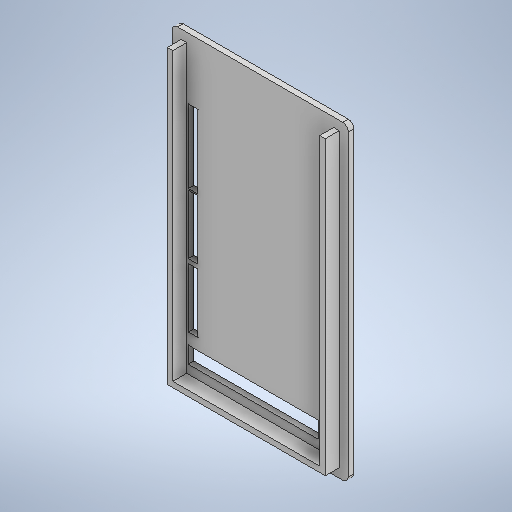
# Autodesk Inventor part: arduino_lid
Saved by Autodesk Inventor 2025 (Build 290162000, 162)
## iProperties
Created: 2025-03-25
Part Number: arduino_lid
Material: Všeobecné
Document SubType Name: Modeling
Designer: lukas
Density: 1 g/cm^3
Appearance: Výchozí
Author: lukas
## iProperties of the stored document arduino_lid_3D tisk.ipt
Created: 2025-03-25
Part Number: arduino_lid_3D tisk
Material: Všeobecné
Document SubType Name: Modeling
Designer: lukas
Density: 1 g/cm^3
Appearance: Výchozí
Author: lukas
Autodesk Inventor part; units mm, degrees
ref_plane "YZ Plane" through (0, 0, 0) normal (1, 0, 0) x (0, 1, 0)
ref_plane "XZ Plane" through (0, 0, 0) normal (0, 1, 0) x (-1, 0, 0)
ref_plane "XY Plane" through (0, 0, 0) normal (0, 0, 1) x (1, 0, 0)
sketch "Náčrt1" plane through (0, 0, 0) normal (0, 1, 0) x (-1, 0, 0)
  line L0 (-6.677663, 17.076554) -> (49.20234, 17.076554)
  line L1 (-9.217661, 14.536556) -> (-9.217661, -88.33345)
  line L2 (-6.677663, -90.873447) -> (49.20234, -90.873447)
  line L3 (51.742337, 14.536556) -> (51.742337, -88.33345)
  line L4 (47.105338, -3.131448) -> (47.105338, -74.251447)
  line L5 (43.679337, -3.131448) -> (47.105338, -3.131448)
  line L6 (43.679337, -29.547447) -> (43.679337, -3.131448)
  line L7 (43.679337, -29.547447) -> (47.105338, -29.547447)
  line L8 (43.679337, -30.055447) -> (47.105338, -30.055447)
  line L9 (43.679337, -51.391447) -> (43.679337, -30.055447)
  line L10 (47.105338, -51.391447) -> (43.679337, -51.391447)
  line L11 (43.679337, -52.915447) -> (47.105338, -52.915447)
  line L12 (43.679337, -74.251447) -> (43.679337, -52.915447)
  line L13 (47.105338, -74.251447) -> (43.679337, -74.251447)
  line L14 (0.434339, -78.380447) -> (47.170339, -78.380447)
  line L15 (47.170339, -84.346448) -> (47.170339, -78.380447)
  line L16 (47.170339, -84.346448) -> (0.434339, -84.346448)
  line L17 (0.434339, -84.346448) -> (0.434339, -78.380447)
  line L18 (-1.154661, -57.995446) -> (-1.154661, -79.331446)
  line L19 (-4.580662, -79.331446) -> (-4.580662, -12.275449)
  line L20 (-1.154661, -79.331446) -> (-4.580662, -79.331446)
  line L21 (-4.580662, -57.995446) -> (-1.154661, -57.995446)
  line L22 (-1.154661, -56.471446) -> (-4.580662, -56.471446)
  line L23 (-1.154661, -35.135447) -> (-1.154661, -56.471446)
  line L24 (-4.580662, -35.135447) -> (-1.154661, -35.135447)
  line L25 (-1.154661, -33.611447) -> (-4.580662, -33.611447)
  line L26 (-1.154661, -12.275449) -> (-1.154661, -33.611447)
  line L27 (-4.580662, -12.275449) -> (-1.154661, -12.275449)
  circle A0 centre (-6.686866, -88.348377) radius 2.522363
  circle A1 centre (49.198008, -88.332369) radius 2.54409
  circle A2 centre (49.211542, 14.551484) radius 2.522363
  circle A3 centre (-6.692632, 14.545779) radius 2.522319
  line L28 (51.742337, 17.076554) -> (-9.217661, 17.076554)
  line L29 (-9.217661, 17.076554) -> (-9.217661, -90.873447)
  line L30 (-9.217661, -90.873447) -> (51.742337, -90.873447)
  line L31 (51.742337, -90.873447) -> (51.742337, 17.076554)
  line L32 (-1.154661, -12.275449) -> (-4.580662, -12.275449)
  line L33 (-4.580662, -12.275449) -> (-4.580662, -33.611447)
  line L34 (-4.580662, -33.611447) -> (-1.154661, -33.611447)
  line L35 (-1.154661, -33.611447) -> (-1.154661, -12.275449)
  line L36 (-4.580662, -35.135447) -> (-1.154661, -35.135447)
  line L37 (-1.154661, -35.135447) -> (-1.154661, -56.471446)
  line L38 (-1.154661, -56.471446) -> (-4.580662, -56.471446)
  line L39 (-4.580662, -56.471446) -> (-4.580662, -35.135447)
  line L40 (-4.580662, -57.995446) -> (-1.154661, -57.995446)
  line L41 (-1.154661, -57.995446) -> (-1.154661, -79.331446)
  line L42 (-1.154661, -79.331446) -> (-4.580662, -79.331446)
  line L43 (-4.580662, -79.331446) -> (-4.580662, -57.995446)
  line L44 (0.434339, -84.346448) -> (47.170339, -84.346448)
  line L45 (47.170339, -84.346448) -> (47.170339, -78.380447)
  line L46 (47.170339, -78.380447) -> (0.434339, -78.380447)
  line L47 (0.434339, -78.380447) -> (0.434339, -84.346448)
  line L48 (43.679337, -74.251447) -> (47.105338, -74.251447)
  line L49 (47.105338, -74.251447) -> (47.105338, -52.915447)
  line L50 (47.105338, -52.915447) -> (43.679337, -52.915447)
  line L51 (43.679337, -52.915447) -> (43.679337, -74.251447)
  line L52 (47.105338, -30.055447) -> (43.679337, -30.055447)
  line L53 (43.679337, -30.055447) -> (43.679337, -51.391447)
  line L54 (43.679337, -51.391447) -> (47.105338, -51.391447)
  line L55 (47.105338, -51.391447) -> (47.105338, -30.055447)
  line L56 (43.679337, -29.547447) -> (47.105338, -29.547447)
  line L57 (47.105338, -29.547447) -> (47.105338, -3.131448)
  line L58 (47.105338, -3.131448) -> (43.679337, -3.131448)
  line L59 (43.679337, -3.131448) -> (43.679337, -29.547447)
  point P0 (0, 0)
  dimension "d0" = 0
  dimension "d1" = 0
  dimension "d2" = 0
  dimension "d3" = 0
  constraints: 64 end point, 16 parallel, 8 horizontal, 8 perpendicular
  measures "d0" distance between parallel lines of L0 L28
  measures "d1" distance between parallel lines of L3 L31
  measures "d2" distance between parallel lines of L30 L2
  measures "d3" distance between parallel lines of L1 L29
sketch "Náčrt1 outline for Vysunutí1" plane through (0, 0, 0) normal (0, 1, 0) x (-1, 0, 0)
  line L0 (51.742337, 14.536556) -> (51.742337, 17.076554)
  line L1 (51.742337, -88.33345) -> (51.742337, 14.536556)
  line L2 (51.742337, 17.076554) -> (49.20234, 17.076554)
  line L3 (51.742337, -90.873447) -> (51.742337, -88.33345)
  line L4 (49.20234, 17.076554) -> (-6.677663, 17.076554)
  line L5 (49.20234, -90.873447) -> (51.742337, -90.873447)
  line L6 (-6.677663, 17.076554) -> (-9.217661, 17.076554)
  line L7 (-6.677663, -90.873447) -> (49.20234, -90.873447)
  line L8 (-9.217661, 17.076554) -> (-9.217661, 14.536556)
  line L9 (-9.217661, -90.873447) -> (-6.677663, -90.873447)
  line L10 (-9.217661, 14.536556) -> (-9.217661, -88.33345)
  line L11 (-9.217661, -88.33345) -> (-9.217661, -90.873447)
  line L12 (-4.580662, -57.995446) -> (-1.154661, -57.995446)
  line L13 (-4.580662, -79.331446) -> (-4.580662, -57.995446)
  line L14 (-1.154661, -79.331446) -> (-4.580662, -79.331446)
  line L15 (-1.154661, -57.995446) -> (-1.154661, -79.331446)
  line L16 (-4.580662, -56.471446) -> (-4.580662, -35.135447)
  line L17 (-1.154661, -56.471446) -> (-4.580662, -56.471446)
  line L18 (-1.154661, -35.135447) -> (-1.154661, -56.471446)
  line L19 (-4.580662, -35.135447) -> (-1.154661, -35.135447)
  line L20 (0.434339, -84.346448) -> (0.434339, -78.380447)
  line L21 (47.170339, -84.346448) -> (0.434339, -84.346448)
  line L22 (47.170339, -78.380447) -> (47.170339, -84.346448)
  line L23 (0.434339, -78.380447) -> (47.170339, -78.380447)
  line L24 (47.105338, -52.915447) -> (47.105338, -74.251447)
  line L25 (43.679337, -52.915447) -> (47.105338, -52.915447)
  line L26 (43.679337, -74.251447) -> (43.679337, -52.915447)
  line L27 (47.105338, -74.251447) -> (43.679337, -74.251447)
  line L28 (-4.580662, -33.611447) -> (-4.580662, -12.275449)
  line L29 (-1.154661, -33.611447) -> (-4.580662, -33.611447)
  line L30 (-1.154661, -12.275449) -> (-1.154661, -33.611447)
  line L31 (-4.580662, -12.275449) -> (-1.154661, -12.275449)
  line L32 (47.105338, -30.055447) -> (47.105338, -51.391447)
  line L33 (43.679337, -30.055447) -> (47.105338, -30.055447)
  line L34 (43.679337, -51.391447) -> (43.679337, -30.055447)
  line L35 (47.105338, -51.391447) -> (43.679337, -51.391447)
  line L36 (47.105338, -29.547447) -> (43.679337, -29.547447)
  line L37 (47.105338, -3.131448) -> (47.105338, -29.547447)
  line L38 (43.679337, -3.131448) -> (47.105338, -3.131448)
  line L39 (43.679337, -29.547447) -> (43.679337, -3.131448)
extrude "Vysunutí1" add sketch "Náčrt1 outline for Vysunutí1" along normal blind 2
sketch "Náčrt2" plane through (0, 2, 0) normal (0, 1, 0) x (1, 0, 0)
  line L0 (-51.742337, -17.076554) -> (9.217661, -17.076554)
  line L1 (9.217661, -17.076554) -> (9.217661, 90.873447)
  line L2 (9.217661, 90.873447) -> (-51.742337, 90.873447)
  line L3 (-51.742337, 90.873447) -> (-51.742337, -17.076554)
  line L4 (-47.105338, 29.547447) -> (-43.679337, 29.547447)
  line L5 (-43.679337, 29.547447) -> (-43.679337, 3.131448)
  line L6 (-43.679337, 3.131448) -> (-47.105338, 3.131448)
  line L7 (-47.105338, 3.131448) -> (-47.105338, 29.547447)
  line L8 (-47.105338, 30.055447) -> (-47.105338, 51.391447)
  line L9 (-47.105338, 51.391447) -> (-43.679337, 51.391447)
  line L10 (-43.679337, 51.391447) -> (-43.679337, 30.055447)
  line L11 (-43.679337, 30.055447) -> (-47.105338, 30.055447)
  line L12 (4.580662, 57.995446) -> (1.154661, 57.995446)
  line L13 (1.154661, 57.995446) -> (1.154661, 79.331446)
  line L14 (1.154661, 79.331446) -> (4.580662, 79.331446)
  line L15 (4.580662, 79.331446) -> (4.580662, 57.995446)
  line L16 (4.580662, 56.471446) -> (4.580662, 35.135447)
  line L17 (4.580662, 35.135447) -> (1.154661, 35.135447)
  line L18 (1.154661, 35.135447) -> (1.154661, 56.471446)
  line L19 (1.154661, 56.471446) -> (4.580662, 56.471446)
  line L20 (4.580662, 33.611447) -> (4.580662, 12.275449)
  line L21 (4.580662, 12.275449) -> (1.154661, 12.275449)
  line L22 (1.154661, 12.275449) -> (1.154661, 33.611447)
  line L23 (1.154661, 33.611447) -> (4.580662, 33.611447)
  line L24 (-0.434339, 84.346448) -> (-0.434339, 78.380447)
  line L25 (-0.434339, 78.380447) -> (-47.170339, 78.380447)
  line L26 (-47.170339, 78.380447) -> (-47.170339, 84.346448)
  line L27 (-47.170339, 84.346448) -> (-0.434339, 84.346448)
  line L28 (-47.105338, 52.915447) -> (-47.105338, 74.251447)
  line L29 (-47.105338, 74.251447) -> (-43.679337, 74.251447)
  line L30 (-43.679337, 74.251447) -> (-43.679337, 52.915447)
  line L31 (-43.679337, 52.915447) -> (-47.105338, 52.915447)
  line L32 (-52.742337, -18.076554) -> (10.217661, -18.076554)
  line L33 (10.217661, -18.076554) -> (10.217661, 91.873447)
  line L34 (10.217661, 91.873447) -> (-52.742337, 91.873447)
  line L35 (-52.742337, 91.873447) -> (-52.742337, -18.076554)
  point P0 (0, 0)
  dimension "d6" = 1
  constraints: 8 end point, 3 other
  measures "d6" distance between parallel lines of L3 L35
extrude "Vysunutí2" add sketch "Náčrt2" against normal up to surface (2 mm away) contours L35 L34 L33 L32
sketch "Náčrt3" plane through (0, 2, 0) normal (0, 1, 0) x (1, 0, 0)
  line L0 (10.217661, -18.076554) -> (10.217661, 91.873447)
  line L1 (10.217661, 91.873447) -> (-52.742337, 91.873447)
  line L2 (-52.742337, 91.873447) -> (-52.742337, -18.076554)
  line L3 (-52.742337, -18.076554) -> (10.217661, -18.076554)
  line L4 (-47.105338, 29.547447) -> (-43.679337, 29.547447)
  line L5 (-43.679337, 29.547447) -> (-43.679337, 3.131448)
  line L6 (-43.679337, 3.131448) -> (-47.105338, 3.131448)
  line L7 (-47.105338, 3.131448) -> (-47.105338, 29.547447)
  line L8 (-47.105338, 30.055447) -> (-47.105338, 51.391447)
  line L9 (-47.105338, 51.391447) -> (-43.679337, 51.391447)
  line L10 (-43.679337, 51.391447) -> (-43.679337, 30.055447)
  line L11 (-43.679337, 30.055447) -> (-47.105338, 30.055447)
  line L12 (4.580662, 57.995446) -> (1.154661, 57.995446)
  line L13 (1.154661, 57.995446) -> (1.154661, 79.331446)
  line L14 (1.154661, 79.331446) -> (4.580662, 79.331446)
  line L15 (4.580662, 79.331446) -> (4.580662, 57.995446)
  line L16 (4.580662, 56.471446) -> (4.580662, 35.135447)
  line L17 (4.580662, 35.135447) -> (1.154661, 35.135447)
  line L18 (1.154661, 35.135447) -> (1.154661, 56.471446)
  line L19 (1.154661, 56.471446) -> (4.580662, 56.471446)
  line L20 (4.580662, 33.611447) -> (4.580662, 12.275449)
  line L21 (4.580662, 12.275449) -> (1.154661, 12.275449)
  line L22 (1.154661, 12.275449) -> (1.154661, 33.611447)
  line L23 (1.154661, 33.611447) -> (4.580662, 33.611447)
  line L24 (-0.434339, 84.346448) -> (-0.434339, 78.380447)
  line L25 (-0.434339, 78.380447) -> (-47.170339, 78.380447)
  line L26 (-47.170339, 78.380447) -> (-47.170339, 84.346448)
  line L27 (-47.170339, 84.346448) -> (-0.434339, 84.346448)
  line L28 (-47.105338, 52.915447) -> (-47.105338, 74.251447)
  line L29 (-47.105338, 74.251447) -> (-43.679337, 74.251447)
  line L30 (-43.679337, 74.251447) -> (-43.679337, 52.915447)
  line L31 (-43.679337, 52.915447) -> (-47.105338, 52.915447)
  line L32 (10.445662, -18.901553) -> (-52.970338, -18.901553)
  line L33 (-52.970338, 92.698447) -> (10.445662, 92.698447)
  line L34 (-52.970338, 92.698447) -> (-52.970338, -18.901553)
  line L35 (10.445662, -18.901553) -> (10.445662, 92.698447)
  line L36 (10.217661, 91.873447) -> (-52.742337, 91.873447)
  line L37 (-21.262338, 91.873447) -> (-21.262338, -18.076554) construction
  line L38 (10.217661, -18.076554) -> (10.217661, 91.873447)
  line L39 (10.217661, 36.898447) -> (-52.742337, 36.898447) construction
  point P0 (0, 0)
  dimension "d10" = 111.6
  dimension "d11" = 63.416
  constraints: 12 end point, 4 midpoint, 2 parallel, 2 other
  measures "d10" distance of L32.start L33.end
  measures "d11" distance of L33.start L33.end
extrude "Vysunutí3" add sketch "Náčrt3" against normal up to surface (2 mm away) contours L32 L34 L33 L35
fillet "Zaoblení1" radius 2 4 edges at (10.4457, 1, -92.6984) (-52.9703, 1, -92.6984) (-52.9703, 1, 18.9016) (10.4457, 1, 18.9016)
sketch "Náčrt4" plane through (0, 2, 0) normal (0, 1, 0) x (1, 0, 0)
  arc A0 (8.445662, -18.901553) -> (10.445662, -16.901553) centre (8.445662, -16.901553) ccw
  line L0 (10.445662, -16.901553) -> (10.445662, 90.698447)
  arc A1 (10.445662, 90.698447) -> (8.445662, 92.698447) centre (8.445662, 90.698447) ccw
  line L1 (8.445662, 92.698447) -> (-50.970338, 92.698447)
  arc A2 (-50.970338, 92.698447) -> (-52.970338, 90.698447) centre (-50.970338, 90.698447) ccw
  line L2 (-52.970338, 90.698447) -> (-52.970338, -16.901553)
  arc A3 (-52.970338, -16.901553) -> (-50.970338, -18.901553) centre (-50.970338, -16.901553) ccw
  line L3 (-50.970338, -18.901553) -> (8.445662, -18.901553)
  line L4 (-47.105338, 29.547447) -> (-43.679337, 29.547447)
  line L5 (-43.679337, 29.547447) -> (-43.679337, 3.131448)
  line L6 (-43.679337, 3.131448) -> (-47.105338, 3.131448)
  line L7 (-47.105338, 3.131448) -> (-47.105338, 29.547447)
  line L8 (-47.105338, 30.055447) -> (-47.105338, 51.391447)
  line L9 (-47.105338, 51.391447) -> (-43.679337, 51.391447)
  line L10 (-43.679337, 51.391447) -> (-43.679337, 30.055447)
  line L11 (-43.679337, 30.055447) -> (-47.105338, 30.055447)
  line L12 (4.580662, 57.995446) -> (1.154661, 57.995446)
  line L13 (1.154661, 57.995446) -> (1.154661, 79.331446)
  line L14 (1.154661, 79.331446) -> (4.580662, 79.331446)
  line L15 (4.580662, 79.331446) -> (4.580662, 57.995446)
  line L16 (4.580662, 56.471446) -> (4.580662, 35.135447)
  line L17 (4.580662, 35.135447) -> (1.154661, 35.135447)
  line L18 (1.154661, 35.135447) -> (1.154661, 56.471446)
  line L19 (1.154661, 56.471446) -> (4.580662, 56.471446)
  line L20 (4.580662, 33.611447) -> (4.580662, 12.275449)
  line L21 (4.580662, 12.275449) -> (1.154661, 12.275449)
  line L22 (1.154661, 12.275449) -> (1.154661, 33.611447)
  line L23 (1.154661, 33.611447) -> (4.580662, 33.611447)
  line L24 (-0.434339, 84.346448) -> (-0.434339, 78.380447)
  line L25 (-0.434339, 78.380447) -> (-47.170339, 78.380447)
  line L26 (-47.170339, 78.380447) -> (-47.170339, 84.346448)
  line L27 (-47.170339, 84.346448) -> (-0.434339, 84.346448)
  line L28 (-47.105338, 52.915447) -> (-47.105338, 74.251447)
  line L29 (-47.105338, 74.251447) -> (-43.679337, 74.251447)
  line L30 (-43.679337, 74.251447) -> (-43.679337, 52.915447)
  line L31 (-43.679337, 52.915447) -> (-47.105338, 52.915447)
  line L32 (7.195662, -15.651553) -> (7.195662, 89.448447)
  line L33 (7.195662, 89.448447) -> (-49.720338, 89.448447)
  line L34 (-49.720338, 89.448447) -> (-49.720338, -15.651553)
  line L35 (5.195662, -15.651553) -> (5.195662, 87.448447)
  line L36 (5.195662, 87.448447) -> (-47.720338, 87.448447)
  line L37 (-47.720338, 87.448447) -> (-47.720338, -15.651553)
  line L38 (7.195662, -15.651553) -> (5.195662, -15.651553)
  line L39 (-47.720338, -15.651553) -> (-49.720338, -15.651553)
  point P0 (0, 0)
  dimension "d17" = 2
  dimension "d18" = 2
  dimension "d19" = 3.25
  dimension "d20" = 2
  constraints: 16 end point, 1 collinear, 1 horizontal, 2 other
  measures "d17" distance between parallel lines of L34 L37
  measures "d18" distance between parallel lines of L32 L35
  measures "d19" distance between parallel lines of L2 L34
  measures "d20" distance between parallel lines of L33 L36
extrude "Vysunutí4" add sketch "Náčrt4" against normal blind 7 contours L38 L35 L36 L37 L39 L34 L33 L32
